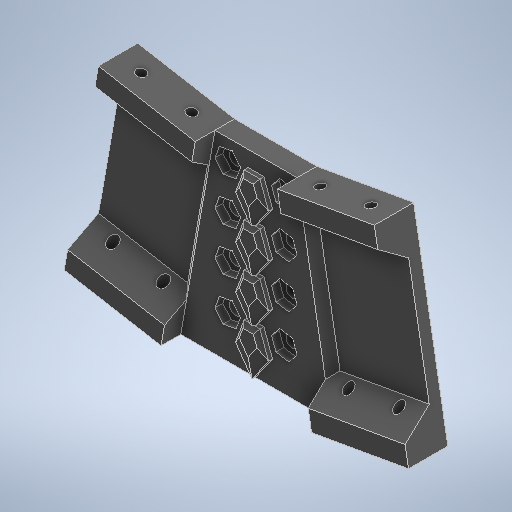
# Autodesk Inventor part: back
Saved by Autodesk Inventor 2026.1 (Build 301233020, 233B)
## iProperties
Created: 2026-02-01
Part Number: back
Material: 一般
Document SubType Name: Modeling
Designer: hibik
Density: 1 g/cm^3
Appearance: 既定
Author: hibik
Autodesk Inventor part; units mm, degrees
ref_plane "YZ Plane" through (0, 0, 0) normal (1, 0, 0) x (0, 1, 0)
ref_plane "作業平面2" through (-4.3412, 24.6202, 0) normal (-0.1736482, 0.9848078, 0) x (0, 0, 1)
ref_plane "作業平面1" through (0, 0, 0) normal (-0.1736482, 0.9848078, 0) x (0, 0, 1)
sketch "スケッチ1" plane through (-4.3412, 24.6202, 0) normal (-0.1736482, 0.9848078, 0) x (0, 0, 1)
  line L0 (0, 15) -> (10, 15)
  line L1 (10, 15) -> (10, 40)
  line L2 (10, 40) -> (0, 40)
  line L3 (0, 40) -> (0, 15)
  point P0 (0, 0)
  dimension "d2" = 10
  dimension "d3" = 25
  dimension "d4" = 15
  constraints: 8 end point, 2 parallel, 1 horizontal, 1 perpendicular, 1 point on line
  measures "d2" distance of L2.end L1.end
  measures "d3" distance of L1.end L0.end
  measures "d4" distance from line of L0 point (0, 0)
extrude "押し出し1" add sketch "スケッチ1" against normal blind 50
mirror "ミラー1" about plane through (0, 0, 0) normal (1, 0, 0) of "押し出し1"
sketch "スケッチ2" plane through (0, 0, 0) normal (0, 0, 1) x (1, 0, 0)
  line L0 (10.4309, 27.2249) -> (19.1133, -22.0155) projected
  line L1 (-10.4309, 27.2249) -> (-19.1133, -22.0155) projected
  line L2 (10.4309, 27.2249) -> (-10.4309, 27.2249)
  line L3 (19.1133, -22.0155) -> (-19.1133, -22.0155)
  point P0 (0, 0)
  constraints: 4 end point, 1 horizontal, 1 parallel
extrude "押し出し2" add sketch "スケッチ2" along normal blind 5
sketch "スケッチ3" plane through (35.0511, 31.5661, 10) normal (0.9848078, 0.1736482, 0) x (0, 0, -1)
  line L0 (0, 3.6226) -> (0, -43.362) projected
  line L1 (0, -5) -> (7, -10)
  line L2 (7, -10) -> (7, -40)
  line L3 (7, -40) -> (0, -45)
  line L4 (10, 0) -> (10, -50) projected
  line L5 (0, 0) -> (10, 0) projected
  line L6 (10, -25) -> (0, -25) construction
  line L7 (0, 0) -> (0, -50) projected
  dimension "d9" = 3
  dimension "d10" = 5
  dimension "d11" = 10
  constraints: 8 end point, 3 point on line, 1 parallel, 1 perpendicular, 1 other
  measures "d9" distance between parallel lines of L4 L2
  measures "d10" distance from line of L5 L1.start
  measures "d11" distance from line of L5 L1.end
extrude "押し出し3" cut sketch "スケッチ3" against normal up to surface (25 mm away)
sketch "スケッチ5" plane through (0, 0, 5) normal (0, 0, 1) x (1, 0, 0)
  line L0 (0, 23.2249) -> (2, 23.2249)
  line L1 (2, 23.2249) -> (4.2012, 17.2249)
  line L2 (4.2012, 17.2249) -> (0, 11.2249)
  line L3 (0, 11.2249) -> (0, 23.2249)
  line L4 (10.4309, 27.2249) -> (-10.4309, 27.2249) projected
  point P0 (0, 0)
  dimension "d19" = 2
  dimension "d20" = 35
  dimension "d21" = 6
  dimension "d22" = 12
  dimension "d23" = 4
  constraints: 8 end point, 1 horizontal, 1 perpendicular, 1 point on line
  measures "d19" distance of L0.start L0.end
  measures "d20" angle of L3 L2
  measures "d21" distance from line of L1.end L0
  measures "d22" distance of L2.end L0.start
  measures "d23" distance between parallel lines of L4 L0
extrude "押し出し4" add sketch "スケッチ5" along normal blind 1
sketch "スケッチ6" plane through (0, 0, 5) normal (0, 0, 1) x (1, 0, 0)
  line L0 (8.3179, 18.6336) -> (5.0756, 19.1968)
  line L1 (5.0756, 19.1968) -> (3.9421, 22.2863)
  line L2 (3.9421, 22.2863) -> (6.051, 24.8127)
  line L3 (6.051, 24.8127) -> (9.2933, 24.2496)
  line L4 (9.2933, 24.2496) -> (10.4268, 21.16)
  line L5 (10.4268, 21.16) -> (8.3179, 18.6336)
  line L6 (4.2012, 17.2249) -> (2, 23.2249) projected
  line L7 (3.1006, 20.2249) -> (7.1845, 21.7232) construction
  point P0 (0, 0)
  dimension "d26" = 5.7
  dimension "d27" = 1.5
  constraints: 14 end point, 1 midpoint, 1 parallel, 1 perpendicular, 13 other
  measures "d26" distance between parallel lines of L0 L3
  measures "d27" distance between parallel lines of L6 L1
extrude "押し出し5" cut sketch "スケッチ6" against normal blind 2
sketch "スケッチ7" plane through (0, 0, 3) normal (0, 0, 1) x (1, 0, 0)
  circle A0 centre (7.1845, 21.7232) radius 2.85
  line L0 (6.051, 24.8127) -> (9.2933, 24.2496) projected
  line L1 (9.2933, 24.2496) -> (10.4268, 21.16) projected
  line L2 (10.4268, 21.16) -> (8.3179, 18.6336) projected
  circle A1 centre (7.1845, 21.7232) radius 1.6
  point P0 (0, 0)
  dimension "d30" = 3.2
  constraints: 3 tangent, 2 centre point, 1 coincident
  measures "d30" diameter of A1
extrude "押し出し6" cut sketch "スケッチ7" against normal through all contours A1
ref_plane "作業平面3" through (0, 0, 7) normal (0, 0, 1) x (1, 0, 0)
sketch "スケッチ8" plane through (0, 0, 7) normal (0, 0, 1) x (1, 0, 0)
  line L0 (0, 22.2249) -> (1.3017, 22.2249)
  line L1 (1.3017, 22.2249) -> (2.2431, 19.6588)
  line L2 (2.2431, 19.6588) -> (0, 16.4553)
  line L3 (0, 16.4553) -> (0, 22.2249)
  line L4 (0, 23.2249) -> (0, 11.2249) construction
  line L5 (2, 23.2249) -> (0, 23.2249) construction
  line L6 (4.2012, 17.2249) -> (2, 23.2249) construction
  line L7 (0, 11.2249) -> (4.2012, 17.2249) construction
  point P0 (0, 0)
  point P1 (0.6508, 22.2249)
  dimension "d34" = 1
  dimension "d35" = 1
  dimension "d36" = 3
  constraints: 8 end point, 3 parallel, 1 collinear, 1 horizontal, 1 midpoint, 1 perpendicular
  measures "d34" distance from line of L5 point (0.651, 22.225)
  measures "d35" distance between parallel lines of L6 L1
  measures "d36" distance between parallel lines of L7 L2
loft "ロフト1" add profiles "スケッチ8" section 2 edges at (2.1006, 14.2249, 6) (3.1006, 20.2249, 6) (1, 23.2249, 6) (0, 17.2249, 6)
pattern_linear "矩形状パターン1" count 4 spacing 11 along (0, -1, 0) of "ロフト1", "押し出し4", "押し出し5", "押し出し6"
mirror "ミラー2" about plane through (0, 0, 0) normal (1, 0, 0) of "ロフト1", "押し出し4", "押し出し5", "押し出し6", "矩形状パターン1", "押し出し3"
chamfer "面取り2" distance 2 angle 45 2 edges at (-14.7721, 2.6047, 3) (14.7721, 2.6047, 3)
sketch "スケッチ10" plane through (-4.3412, 24.6202, 0) normal (-0.1736482, 0.9848078, 0) x (0.9848078, 0.1736482, 0)
  circle A0 centre (21, -5) radius 1.25
  circle A1 centre (34, -5) radius 1.25
  line L0 (40, -10) -> (40, 0) projected
  line L1 (15, -5) -> (15, -10) projected
  point P0 (0, 0)
  point P1 (40, -5)
  dimension "d47" = 2.5
  dimension "d48" = 2.5
  dimension "d49" = 6
  dimension "d50" = 6
  constraints: 2 centre point, 2 horizontal alignment, 1 midpoint
  measures "d47" diameter of A0
  measures "d48" diameter of A1
  measures "d49" distance from line of L0 A1.centre
  measures "d50" distance from line of L1 A0.centre
extrude "押し出し7" cut sketch "スケッチ10" against normal through all
mirror "ミラー3" about plane through (0, 0, 0) normal (1, 0, 0) of "押し出し7"
ref_plane "作業平面4" through (0, 0, 0) normal (1, 0, 0) x (0, 1, 0)
equation "\"d19\" = 0.166667 * d22"
equation "\"d21\" = 0.5 * d22"
equation "\"d23\" = 0.333333 * d22"
